Autodesk Fusion 360 part; units mm, degrees
note: some values were not read from the file. Set by a fixed rule: which sketch regions a step uses.
(part 2 of 2)
sketch "Sketch5" plane through (0, 0, 0) normal (0, 0, 1) x (1, 0, 0)
  line L0 (-28.8618, -57.7236) -> (1022.0897, -57.7236)
  line L1 (1022.0897, -57.7236) -> (1022.0897, -272.5388)
  line L2 (1022.0897, -272.5388) -> (-28.8618, -272.5388)
  line L3 (-28.8618, -272.5388) -> (-28.8618, -57.7236)
  line L4 (199.3413, -86.9336) -> (377.0355, -86.9336)
  line L5 (377.0355, -86.9336) -> (377.0355, -237.8519)
  line L6 (377.0355, -237.8519) -> (199.3413, -237.8519)
  line L7 (199.3413, -237.8519) -> (199.3413, -86.9336)
  spline S0 degree 3 poles (267.5473, -188.3142) (266.8998, -187.7866) (266.0771, -187.5231) (265.2567, -187.3679) knots 0 0 0 0 1 1 1 1
  spline S1 degree 3 poles (265.2567, -187.3679) (263.5948, -187.0539) (262.7928, -187.5736) (262.4666, -188.5278) knots 0 0 0 0 1 1 1 1
  spline S2 degree 3 poles (262.4666, -188.5278) (261.4698, -191.4391) (265.1758, -197.3711) (261.7953, -199.3136) knots 0 0 0 0 1 1 1 1
  spline S3 degree 3 poles (261.7953, -199.3136) (261.1984, -199.6568) (260.504, -199.7943) (259.8961, -200.1175) knots 0 0 0 0 1 1 1 1
  spline S4 degree 3 poles (259.8961, -200.1175) (259.2237, -200.4753) (258.6608, -201.082) (258.4703, -201.8196) knots 0 0 0 0 1 1 1 1
  spline S5 degree 3 poles (258.4703, -201.8196) (258.2786, -202.5571) (258.5104, -203.4164) (259.1172, -203.8764) knots 0 0 0 0 1 1 1 1
  spline S6 degree 3 poles (259.1172, -203.8764) (259.5863, -204.2318) (260.201, -204.3188) (260.7876, -204.3681) knots 0 0 0 0 1 1 1 1
  spline S7 degree 3 poles (260.7876, -204.3681) (265.3724, -204.7539) (268.5203, -204.1558) (269.4021, -199.0495) knots 0 0 0 0 1 1 1 1
  spline S8 degree 3 poles (269.4021, -199.0495) (269.9376, -195.955) (270.1658, -192.6087) (268.7102, -189.8258) knots 0 0 0 0 1 1 1 1
  spline S9 degree 3 poles (268.7102, -189.8258) (268.4132, -189.2587) (268.0439, -188.7183) (267.5473, -188.3142) knots 0 0 0 0 1 1 1 1
  spline S10 degree 3 poles (312.6049, -189.9938) (311.9453, -189.4832) (311.1152, -189.2398) (310.2912, -189.1059) knots 0 0 0 0 1 1 1 1
  spline S11 degree 3 poles (310.2912, -189.1059) (308.6233, -188.8345) (307.834, -189.3731) (307.5309, -190.3364) knots 0 0 0 0 1 1 1 1
  spline S12 degree 3 poles (307.5309, -190.3364) (306.6096, -193.2708) (310.4641, -199.1073) (307.1335, -201.135) knots 0 0 0 0 1 1 1 1
  spline S13 degree 3 poles (307.1335, -201.135) (306.5451, -201.4928) (305.855, -201.6486) (305.255, -201.9869) knots 0 0 0 0 1 1 1 1
  spline S14 degree 3 poles (305.255, -201.9869) (304.5917, -202.3612) (304.0452, -202.9825) (303.8736, -203.7249) knots 0 0 0 0 1 1 1 1
  spline S15 degree 3 poles (303.8736, -203.7249) (303.7008, -204.4667) (303.9527, -205.3199) (304.5722, -205.7647) knots 0 0 0 0 1 1 1 1
  spline S16 degree 3 poles (304.5722, -205.7647) (305.0499, -206.108) (305.6663, -206.1792) (306.2542, -206.2132) knots 0 0 0 0 1 1 1 1
  spline S17 degree 3 poles (306.2542, -206.2132) (310.8475, -206.4834) (313.9784, -205.8055) (314.7312, -200.6792) knots 0 0 0 0 1 1 1 1
  spline S18 degree 3 poles (314.7312, -200.6792) (315.1882, -197.5713) (315.3318, -194.2213) (313.8056, -191.4756) knots 0 0 0 0 1 1 1 1
  spline S19 degree 3 poles (313.8056, -191.4756) (313.4946, -190.9163) (313.1118, -190.3851) (312.6049, -189.9938) knots 0 0 0 0 1 1 1 1
  line L8 (341.835, -190.3857) -> (341.2265, -189.7771)
  spline S20 degree 2 poles (341.2265, -189.7771) (340.0429, -189.6524) (339.4051, -189.2252) knots 0 0 0 1 1 1
  spline S21 degree 3 poles (339.4051, -189.2252) (338.7661, -188.7986) (338.1399, -188.2953) (337.3841, -188.1602) knots 0 0 0 0 1 1 1 1
  spline S22 degree 3 poles (337.3841, -188.1602) (337.49, -189.3177) (337.7182, -190.4642) (338.0645, -191.5754) knots 0 0 0 0 1 1 1 1
  spline S23 degree 3 poles (338.0645, -191.5754) (335.808, -191.3916) (334.0183, -189.6548) (332.5413, -187.9387) knots 0 0 0 0 1 1 1 1
  spline S24 degree 3 poles (332.5413, -187.9387) (332.0478, -187.3649) (331.4655, -186.6413) (330.7182, -186.6316) knots 0 0 0 0 1 1 1 1
  spline S25 degree 3 poles (330.7182, -186.6316) (330.6567, -187.1318) (333.484, -192.6695) (332.3241, -192.4103) knots 0 0 0 0 1 1 1 1
  spline S26 degree 2 poles (332.3241, -192.4103) (330.6555, -192.0366) (318.896, -185.9001) knots 0 0 0 1 1 1
  spline S27 degree 2 poles (318.896, -185.9001) (321.626, -194.0418) (319.3658, -193.1856) knots 0 0 0 1 1 1
  spline S28 degree 2 poles (319.3658, -193.1856) (317.1057, -192.3287) (308.1388, -184.2784) knots 0 0 0 1 1 1
  spline S29 degree 2 poles (308.1388, -184.2784) (307.8297, -191.9143) (306.1069, -191.004) knots 0 0 0 1 1 1
  spline S30 degree 2 poles (306.1069, -191.004) (304.3847, -190.093) (295.8189, -180.6435) knots 0 0 0 1 1 1
  spline S31 degree 2 poles (295.8189, -180.6435) (295.1081, -189.6779) (292.2291, -188.0702) knots 0 0 0 1 1 1
  spline S32 degree 2 poles (292.2291, -188.0702) (289.3495, -186.4618) (282.7693, -175.1813) knots 0 0 0 1 1 1
  spline S33 degree 2 poles (282.7693, -175.1813) (288.6101, -163.1796) (279.7388, -164.0821) knots 0 0 0 1 1 1
  spline S34 degree 3 poles (279.7388, -164.0821) (275.6281, -164.5008) (272.1966, -166.0489) (270.29, -169.9241) knots 0 0 0 0 1 1 1 1
  spline S35 degree 3 poles (270.29, -169.9241) (268.8027, -168.3297) (266.5115, -167.639) (264.336, -167.7771) knots 0 0 0 0 1 1 1 1
  spline S36 degree 3 poles (264.336, -167.7771) (262.284, -167.9865) (260.8972, -168.5384) (259.032, -169.4464) knots 0 0 0 0 1 1 1 1
  spline S37 degree 3 poles (259.032, -169.4464) (258.5963, -169.6581) (258.0893, -169.873) (257.6463, -169.6776) knots 0 0 0 0 1 1 1 1
  spline S38 degree 3 poles (257.6463, -169.6776) (257.3554, -169.5498) (257.165, -169.2735) (256.9648, -169.0277) knots 0 0 0 0 1 1 1 1
  spline S39 degree 3 poles (256.9648, -169.0277) (256.2101, -168.0985) (255.1032, -167.4455) (253.9147, -167.3073) knots 0 0 0 0 1 1 1 1
  spline S40 degree 3 poles (253.9147, -167.3073) (252.7135, -167.168) (250.4527, -167.7601) (250.0797, -169.1476) knots 0 0 0 0 1 1 1 1
  spline S41 degree 3 poles (250.0797, -169.1476) (250.5264, -167.4856) (251.1714, -165.1196) (250.4655, -163.4303) knots 0 0 0 0 1 1 1 1
  spline S42 degree 3 poles (250.4655, -163.4303) (250.3365, -163.1212) (250.1187, -162.8479) (249.8479, -162.6264) knots 0 0 0 0 1 1 1 1
  spline S43 degree 3 poles (249.8479, -162.6264) (248.9935, -161.9254) (247.6096, -161.7349) (246.8131, -162.5382) knots 0 0 0 0 1 1 1 1
  spline S44 degree 3 poles (246.8131, -162.5382) (246.185, -163.1717) (246.1564, -164.2086) (246.4528, -165.0503) knots 0 0 0 0 1 1 1 1
  spline S45 degree 3 poles (246.4528, -165.0503) (246.7492, -165.8913) (247.3108, -166.6081) (247.766, -167.3755) knots 0 0 0 0 1 1 1 1
  spline S46 degree 3 poles (247.766, -167.3755) (248.747, -169.0326) (249.6269, -171.6176) (249.0403, -173.5285) knots 0 0 0 0 1 1 1 1
  spline S47 degree 3 poles (249.0403, -173.5285) (248.4969, -175.2969) (246.883, -176.8462) (245.2674, -177.6386) knots 0 0 0 0 1 1 1 1
  spline S48 degree 3 poles (245.2674, -177.6386) (238.2831, -181.0653) (232.6152, -184.0861) (235.577, -186.5007) knots 0 0 0 0 1 1 1 1
  spline S49 degree 3 poles (235.577, -186.5007) (238.5387, -188.9154) (253.3829, -190.6638) (259.2194, -191.9721) knots 0 0 0 0 1 1 1 1
  spline S50 degree 3 poles (259.2194, -191.9721) (265.0559, -193.2793) (270.7872, -196.2271) (282.1925, -198.8687) knots 0 0 0 0 1 1 1 1
  spline S51 degree 3 poles (282.1925, -198.8687) (293.5965, -201.5104) (328.2505, -200.429) (337.1937, -194.9017) knots 0 0 0 0 1 1 1 1
  spline S52 degree 3 poles (337.1937, -194.9017) (339.2347, -193.642) (343.1957, -194.1337) (342.1393, -191.2985) knots 0 0 0 0 1 1 1 1
  line L9 (342.1393, -191.2985) -> (341.835, -190.3857)
  spline S53 degree 3 poles (278.798, -190.7575) (278.1505, -190.2305) (277.3278, -189.967) (276.5074, -189.8118) knots 0 0 0 0 1 1 1 1
  spline S54 degree 3 poles (276.5074, -189.8118) (274.8467, -189.4978) (274.0441, -190.0163) (273.7173, -190.9717) knots 0 0 0 0 1 1 1 1
  spline S55 degree 3 poles (273.7173, -190.9717) (272.7211, -193.8817) (276.4265, -199.8138) (273.0461, -201.7575) knots 0 0 0 0 1 1 1 1
  spline S56 degree 3 poles (273.0461, -201.7575) (272.4491, -202.0995) (271.7554, -202.2382) (271.1468, -202.5614) knots 0 0 0 0 1 1 1 1
  spline S57 degree 3 poles (271.1468, -202.5614) (270.4744, -202.9186) (269.9127, -203.5259) (269.721, -204.2635) knots 0 0 0 0 1 1 1 1
  spline S58 degree 3 poles (269.721, -204.2635) (269.5299, -205.001) (269.7605, -205.8597) (270.3679, -206.3197) knots 0 0 0 0 1 1 1 1
  spline S59 degree 3 poles (270.3679, -206.3197) (270.8365, -206.6757) (271.4517, -206.7628) (272.0383, -206.812) knots 0 0 0 0 1 1 1 1
  spline S60 degree 3 poles (272.0383, -206.812) (276.6231, -207.1979) (279.7711, -206.5991) (280.6535, -201.4934) knots 0 0 0 0 1 1 1 1
  spline S61 degree 3 poles (280.6535, -201.4934) (281.1884, -198.3983) (281.4172, -195.0526) (279.9609, -192.2697) knots 0 0 0 0 1 1 1 1
  spline S62 degree 3 poles (279.9609, -192.2697) (279.664, -191.7026) (279.2946, -191.1616) (278.798, -190.7575) knots 0 0 0 0 1 1 1 1
  spline S63 degree 3 poles (327.0627, -190.6504) (326.4024, -190.1398) (325.5729, -189.897) (324.7496, -189.7625) knots 0 0 0 0 1 1 1 1
  spline S64 degree 3 poles (324.7496, -189.7625) (323.0804, -189.4905) (322.2911, -190.0297) (321.9893, -190.9924) knots 0 0 0 0 1 1 1 1
  spline S65 degree 3 poles (321.9893, -190.9924) (321.0667, -193.9274) (324.9212, -199.7639) (321.5906, -201.7916) knots 0 0 0 0 1 1 1 1
  spline S66 degree 3 poles (321.5906, -201.7916) (321.0034, -202.1494) (320.3121, -202.3058) (319.7133, -202.6435) knots 0 0 0 0 1 1 1 1
  spline S67 degree 3 poles (319.7133, -202.6435) (319.0494, -203.0184) (318.5023, -203.6391) (318.3307, -204.3815) knots 0 0 0 0 1 1 1 1
  spline S68 degree 3 poles (318.3307, -204.3815) (318.1579, -205.1239) (318.4104, -205.9765) (319.0293, -206.4214) knots 0 0 0 0 1 1 1 1
  spline S69 degree 3 poles (319.0293, -206.4214) (319.507, -206.7646) (320.1235, -206.8358) (320.7113, -206.8705) knots 0 0 0 0 1 1 1 1
  spline S70 degree 3 poles (320.7113, -206.8705) (325.3046, -207.14) (328.4367, -206.4615) (329.1895, -201.3352) knots 0 0 0 0 1 1 1 1
  spline S71 degree 3 poles (329.1895, -201.3352) (329.6453, -198.2279) (329.7889, -194.8773) (328.2633, -192.1328) knots 0 0 0 0 1 1 1 1
  spline S72 degree 3 poles (328.2633, -192.1328) (327.9517, -191.5729) (327.569, -191.0411) (327.0627, -190.6504) knots 0 0 0 0 1 1 1 1
  line L10 (614.3667, -86.9336) -> (792.0609, -86.9336)
  line L11 (792.0609, -86.9336) -> (792.0609, -237.8519)
  line L12 (792.0609, -237.8519) -> (614.3667, -237.8519)
  line L13 (614.3667, -237.8519) -> (614.3667, -86.9336)
  spline S73 degree 3 poles (661.9365, -162.4475) (662.7458, -161.7508) (664.0542, -161.9528) (664.8757, -162.6264) knots 0 0 0 0 1 1 1 1
  spline S74 degree 3 poles (664.8757, -162.6264) (665.1434, -162.8479) (665.3626, -163.1212) (665.4903, -163.4303) knots 0 0 0 0 1 1 1 1
  spline S75 degree 3 poles (665.4903, -163.4303) (666.1902, -165.1069) (665.5634, -167.4491) (665.113, -169.1092) knots 0 0 0 0 1 1 1 1
  line L14 (665.113, -169.1092) -> (665.107, -169.147)
  spline S76 degree 3 poles (665.107, -169.147) (665.4782, -167.7601) (667.7419, -167.168) (668.9408, -167.3073) knots 0 0 0 0 1 1 1 1
  spline S77 degree 3 poles (668.9408, -167.3073) (670.1274, -167.4455) (671.2349, -168.0985) (671.9895, -169.0277) knots 0 0 0 0 1 1 1 1
  spline S78 degree 3 poles (671.9895, -169.0277) (672.02, -169.0606) (672.0443, -169.0946) (672.0686, -169.1287) knots 0 0 0 0 1 1 1 1
  spline S79 degree 3 poles (672.0686, -169.1287) (672.2451, -169.3454) (672.4216, -169.5675) (672.6712, -169.6776) knots 0 0 0 0 1 1 1 1
  spline S80 degree 3 poles (672.6712, -169.6776) (673.1154, -169.873) (673.6204, -169.6581) (674.0586, -169.4464) knots 0 0 0 0 1 1 1 1
  spline S81 degree 3 poles (674.0586, -169.4464) (675.9207, -168.5384) (677.3082, -167.9865) (679.359, -167.7771) knots 0 0 0 0 1 1 1 1
  spline S82 degree 3 poles (679.359, -167.7771) (681.5376, -167.639) (683.8257, -168.3297) (685.3166, -169.9241) knots 0 0 0 0 1 1 1 1
  spline S83 degree 3 poles (685.3166, -169.9241) (687.2213, -166.0489) (690.6535, -164.5008) (694.7612, -164.0821) knots 0 0 0 0 1 1 1 1
  spline S84 degree 2 poles (694.7612, -164.0821) (703.6337, -163.1796) (697.7917, -175.1813) knots 0 0 0 1 1 1
  spline S85 degree 2 poles (697.7917, -175.1813) (704.3762, -186.4618) (707.2546, -188.0702) knots 0 0 0 1 1 1
  spline S86 degree 2 poles (707.2546, -188.0702) (710.1329, -189.6779) (710.845, -180.6435) knots 0 0 0 1 1 1
  spline S87 degree 2 poles (710.845, -180.6435) (719.4071, -190.093) (721.1354, -191.004) knots 0 0 0 1 1 1
  spline S88 degree 2 poles (721.1354, -191.004) (722.8576, -191.9143) (723.1618, -184.2784) knots 0 0 0 1 1 1
  spline S89 degree 2 poles (723.1618, -184.2784) (732.1317, -192.3287) (734.3894, -193.1856) knots 0 0 0 1 1 1
  spline S90 degree 2 poles (734.3894, -193.1856) (736.6532, -194.0418) (733.9208, -185.9001) knots 0 0 0 1 1 1
  spline S91 degree 2 poles (733.9208, -185.9001) (745.684, -192.0366) (747.3514, -192.4103) knots 0 0 0 1 1 1
  spline S92 degree 3 poles (747.3514, -192.4103) (748.1181, -192.5825) (747.1323, -190.1982) (746.3959, -188.4304) knots 0 0 0 0 1 1 1 1
  line L15 (746.3959, -188.4304) -> (746.3959, -188.4298)
  line L16 (746.3959, -188.4298) -> (746.3959, -188.4292)
  spline S93 degree 3 poles (746.3959, -188.4292) (746.0308, -187.5353) (745.7204, -186.7995) (745.7448, -186.6316) knots 0 0 0 0 1 1 1 1
  spline S94 degree 3 poles (745.7448, -186.6316) (746.4568, -186.6407) (747.0166, -187.2967) (747.4974, -187.8548) knots 0 0 0 0 1 1 1 1
  line L17 (747.4974, -187.8548) -> (747.5643, -187.9387)
  spline S95 degree 3 poles (747.5643, -187.9387) (749.0431, -189.6548) (750.8322, -191.3916) (753.0899, -191.5754) knots 0 0 0 0 1 1 1 1
  spline S96 degree 3 poles (753.0899, -191.5754) (752.743, -190.4642) (752.5179, -189.3177) (752.4083, -188.1602) knots 0 0 0 0 1 1 1 1
  spline S97 degree 3 poles (752.4083, -188.1602) (753.0473, -188.2746) (753.595, -188.6501) (754.1305, -189.0213) knots 0 0 0 0 1 1 1 1
  spline S98 degree 3 poles (754.1305, -189.0213) (754.2278, -189.0901) (754.3313, -189.1589) (754.4287, -189.2252) knots 0 0 0 0 1 1 1 1
  spline S99 degree 3 poles (754.4287, -189.2252) (754.7391, -189.4321) (755.1772, -189.5684) (755.5423, -189.6536) knots 0 0 0 0 1 1 1 1
  spline S100 degree 3 poles (755.5423, -189.6536) (755.2259, -187.8657) (753.3638, -186.3462) (751.9519, -185.1924) knots 0 0 0 0 1 1 1 1
  spline S101 degree 3 poles (751.9519, -185.1924) (749.9133, -183.5244) (748.8058, -182.6213) (754.6356, -182.7789) knots 0 0 0 0 1 1 1 1
  spline S102 degree 3 poles (754.6356, -182.7789) (754.4165, -180.9618) (752.4205, -180.0301) (750.4002, -179.0851) knots 0 0 0 0 1 1 1 1
  spline S103 degree 3 poles (750.4002, -179.0851) (748.5563, -178.2228) (746.688, -177.3483) (746.116, -175.7807) knots 0 0 0 0 1 1 1 1
  spline S104 degree 3 poles (746.116, -175.7807) (747.3209, -176.5225) (748.3859, -176.0229) (749.463, -175.5166) knots 0 0 0 0 1 1 1 1
  spline S105 degree 3 poles (749.463, -175.5166) (750.5219, -175.0218) (751.5868, -174.521) (752.81, -175.1721) knots 0 0 0 0 1 1 1 1
  spline S106 degree 3 poles (752.81, -175.1721) (752.67, -172.4982) (750.0776, -170.4091) (747.6739, -168.4709) knots 0 0 0 0 1 1 1 1
  spline S107 degree 3 poles (747.6739, -168.4709) (746.7793, -167.7497) (745.9091, -167.0499) (745.2032, -166.3483) knots 0 0 0 0 1 1 1 1
  spline S108 degree 3 poles (745.2032, -166.3483) (744.6008, -165.7513) (743.9861, -165.3229) (743.4262, -164.9292) knots 0 0 0 0 1 1 1 1
  spline S109 degree 3 poles (743.4262, -164.9292) (742.2213, -164.0918) (741.2538, -163.4145) (741.126, -161.6157) knots 0 0 0 0 1 1 1 1
  line L18 (741.126, -161.6157) -> (748.0633, -162.2948)
  spline S110 degree 3 poles (748.0633, -162.2948) (745.2276, -158.6618) (741.0408, -156.1059) (736.5132, -155.2387) knots 0 0 0 0 1 1 1 1
  spline S111 degree 3 poles (736.5132, -155.2387) (735.7282, -155.0896) (734.6937, -154.6442) (734.8945, -153.8738) knots 0 0 0 0 1 1 1 1
  spline S112 degree 3 poles (734.8945, -153.8738) (735.0527, -153.3011) (735.7952, -153.1679) (736.3854, -153.1557) knots 0 0 0 0 1 1 1 1
  spline S113 degree 3 poles (736.3854, -153.1557) (738.844, -153.104) (741.3085, -153.2239) (743.7549, -153.5154) knots 0 0 0 0 1 1 1 1
  spline S114 degree 3 poles (743.7549, -153.5154) (741.6797, -150.9035) (738.2597, -149.7473) (734.9493, -149.3219) knots 0 0 0 0 1 1 1 1
  spline S115 degree 3 poles (734.9493, -149.3219) (733.5131, -149.1369) (732.0587, -149.0645) (730.6104, -148.9921) knots 0 0 0 0 1 1 1 1
  spline S116 degree 3 poles (730.6104, -148.9921) (728.7239, -148.8983) (726.8435, -148.8046) (724.9875, -148.4645) knots 0 0 0 0 1 1 1 1
  spline S117 degree 3 poles (724.9875, -148.4645) (724.6466, -147.5103) (725.955, -146.8512) (726.953, -146.7088) knots 0 0 0 0 1 1 1 1
  spline S118 degree 3 poles (726.953, -146.7088) (729.6246, -146.3291) (732.3386, -146.2323) (735.0345, -146.4204) knots 0 0 0 0 1 1 1 1
  spline S119 degree 3 poles (735.0345, -146.4204) (735.3022, -145.2727) (734.5355, -144.0799) (733.5192, -143.4848) knots 0 0 0 0 1 1 1 1
  spline S120 degree 3 poles (733.5192, -143.4848) (732.5029, -142.8902) (731.2859, -142.7612) (730.1052, -142.6687) knots 0 0 0 0 1 1 1 1
  spline S121 degree 3 poles (730.1052, -142.6687) (726.1497, -142.3571) (722.1699, -142.3042) (718.2022, -142.5129) knots 0 0 0 0 1 1 1 1
  spline S122 degree 3 poles (718.2022, -142.5129) (718.3848, -141.008) (720.2104, -140.4299) (721.6891, -140.0818) knots 0 0 0 0 1 1 1 1
  spline S123 degree 3 poles (721.6891, -140.0818) (723.1679, -139.7349) (724.957, -138.7917) (724.7197, -137.2941) knots 0 0 0 0 1 1 1 1
  spline S124 degree 3 poles (724.7197, -137.2941) (717.8127, -137.3379) (710.918, -138.3548) (704.2971, -140.3033) knots 0 0 0 0 1 1 1 1
  spline S125 degree 3 poles (704.2971, -140.3033) (703.725, -139.2396) (704.7108, -138.0219) (705.648, -137.2582) knots 0 0 0 0 1 1 1 1
  spline S126 degree 3 poles (705.648, -137.2582) (706.5913, -136.4957) (707.6805, -135.4471) (707.3215, -134.2927) knots 0 0 0 0 1 1 1 1
  spline S127 degree 3 poles (707.3215, -134.2927) (703.8285, -133.7791) (700.2989, -134.9305) (697.1162, -136.4494) knots 0 0 0 0 1 1 1 1
  spline S128 degree 3 poles (697.1162, -136.4494) (696.0269, -136.9691) (694.956, -137.5338) (693.8849, -138.0979) knots 0 0 0 0 1 1 1 1
  spline S129 degree 3 poles (693.8849, -138.0979) (691.828, -139.1842) (689.7773, -140.2698) (687.5804, -141.0305) knots 0 0 0 0 1 1 1 1
  spline S130 degree 3 poles (687.5804, -141.0305) (687.7629, -139.3564) (688.262, -137.7176) (689.0409, -136.2236) knots 0 0 0 0 1 1 1 1
  spline S131 degree 3 poles (689.0409, -136.2236) (685.2253, -137.2728) (681.8053, -139.6887) (679.5355, -142.931) knots 0 0 0 0 1 1 1 1
  spline S132 degree 3 poles (679.5355, -142.931) (678.6348, -144.2193) (677.1804, -145.8447) (675.8416, -145.0171) knots 0 0 0 0 1 1 1 1
  line L19 (675.8416, -145.0171) -> (677.0891, -139.7325)
  spline S133 degree 3 poles (677.0891, -139.7325) (676.0485, -139.4775) (675.1235, -140.4043) (674.4724, -141.2538) knots 0 0 0 0 1 1 1 1
  spline S134 degree 3 poles (674.4724, -141.2538) (671.8131, -144.7256) (669.5311, -148.4809) (667.6628, -152.4352) knots 0 0 0 0 1 1 1 1
  spline S135 degree 3 poles (667.6628, -152.4352) (666.7926, -152.7541) (665.9954, -151.753) (665.7885, -150.8469) knots 0 0 0 0 1 1 1 1
  spline S136 degree 3 poles (665.7885, -150.8469) (665.746, -150.6497) (665.7094, -150.4459) (665.6729, -150.2414) knots 0 0 0 0 1 1 1 1
  spline S137 degree 3 poles (665.6729, -150.2414) (665.5451, -149.5032) (665.4112, -148.7529) (664.8513, -148.2825) knots 0 0 0 0 1 1 1 1
  spline S138 degree 3 poles (664.8513, -148.2825) (663.2691, -152.0232) (662.2286, -155.9939) (661.7722, -160.0316) knots 0 0 0 0 1 1 1 1
  line L20 (661.7722, -160.0316) -> (661.7722, -161.1757)
  spline S139 degree 2 poles (661.7722, -161.1757) (661.7356, -161.4939) (661.9365, -162.4475) knots 0 0 0 1 1 1
  line L21 (-8.1714, -88.1507) -> (169.5228, -88.1507)
  line L22 (169.5228, -88.1507) -> (169.5228, -239.069)
  line L23 (169.5228, -239.069) -> (-8.1714, -239.069)
  line L24 (-8.1714, -239.069) -> (-8.1714, -88.1507)
  spline S140 degree 3 poles (115.4575, -199.9921) (115.4946, -201.2524) (115.1788, -202.3387) (114.078, -203.0087) knots 0 0 0 0 1 1 1 1
  spline S141 degree 3 poles (114.078, -203.0087) (113.7682, -203.1973) (113.4299, -203.33) (113.0915, -203.4626) knots 0 0 0 0 1 1 1 1
  spline S142 degree 3 poles (113.0915, -203.4626) (112.7878, -203.5813) (112.4836, -203.7006) (112.2006, -203.8606) knots 0 0 0 0 1 1 1 1
  spline S143 degree 3 poles (112.2006, -203.8606) (111.5367, -204.2355) (110.9896, -204.8562) (110.818, -205.5986) knots 0 0 0 0 1 1 1 1
  spline S144 degree 3 poles (110.818, -205.5986) (110.6452, -206.341) (110.8977, -207.1936) (111.5166, -207.6384) knots 0 0 0 0 1 1 1 1
  spline S145 degree 3 poles (111.5166, -207.6384) (111.9943, -207.9817) (112.6114, -208.0529) (113.1986, -208.0875) knots 0 0 0 0 1 1 1 1
  spline S146 degree 3 poles (113.1986, -208.0875) (117.7919, -208.3571) (120.924, -207.6786) (121.6768, -202.5522) knots 0 0 0 0 1 1 1 1
  spline S147 degree 3 poles (121.6768, -202.5522) (121.8557, -201.3309) (121.9872, -200.0718) (121.9872, -198.8261) knots 0 0 0 0 1 1 1 1
  spline S148 degree 3 poles (121.9872, -198.8261) (125.2745, -198.0862) (127.9557, -197.1849) (129.681, -196.1188) knots 0 0 0 0 1 1 1 1
  spline S149 degree 3 poles (129.681, -196.1188) (130.3485, -195.7068) (131.2224, -195.4816) (132.0579, -195.2668) knots 0 0 0 0 1 1 1 1
  spline S150 degree 3 poles (132.0579, -195.2668) (133.7771, -194.8244) (135.3374, -194.4227) (134.6266, -192.5156) knots 0 0 0 0 1 1 1 1
  line L25 (134.6266, -192.5156) -> (134.5073, -192.1584)
  spline S151 degree 3 poles (134.5073, -192.1584) (135.8345, -192.0811) (138.0022, -191.9082) (138.9131, -191.5711) knots 0 0 0 0 1 1 1 1
  spline S152 degree 2 poles (138.9131, -191.5711) (140.2787, -191.0654) (138.2182, -186.0936) knots 0 0 0 1 1 1
  spline S153 degree 2 poles (138.2182, -186.0936) (142.5121, -187.301) (144.5056, -184.9362) knots 0 0 0 1 1 1
  spline S154 degree 2 poles (144.5056, -184.9362) (146.5211, -182.5458) (135.7889, -175.2555) knots 0 0 0 1 1 1
  spline S155 degree 2 poles (135.7889, -175.2555) (141.7781, -175.4058) (144.1326, -172.9108) knots 0 0 0 1 1 1
  spline S156 degree 2 poles (144.1326, -172.9108) (146.5163, -170.3841) (132.0634, -165.6984) knots 0 0 0 1 1 1
  spline S157 degree 2 poles (132.0634, -165.6984) (139.6477, -164.0109) (140.8611, -160.5696) knots 0 0 0 1 1 1
  spline S158 degree 2 poles (140.8611, -160.5696) (142.0849, -157.0984) (126.9297, -155.0848) knots 0 0 0 1 1 1
  spline S159 degree 2 poles (126.9297, -155.0848) (136.723, -151.3143) (136.5216, -148.1182) knots 0 0 0 1 1 1
  spline S160 degree 2 poles (136.5216, -148.1182) (136.3195, -144.9136) (119.0631, -147.321) knots 0 0 0 1 1 1
  spline S161 degree 2 poles (119.0631, -147.321) (128.4517, -142.0188) (126.9163, -139.5256) knots 0 0 0 1 1 1
  spline S162 degree 2 poles (126.9163, -139.5256) (125.3871, -137.0427) (106.7322, -140.6264) knots 0 0 0 1 1 1
  spline S163 degree 2 poles (106.7322, -140.6264) (119.1501, -132.9339) (116.8486, -129.6459) knots 0 0 0 1 1 1
  spline S164 degree 2 poles (116.8486, -129.6459) (113.7731, -125.2529) (95.0787, -135.7636) knots 0 0 0 1 1 1
  spline S165 degree 2 poles (95.0787, -135.7636) (105.7062, -126.7487) (103.2623, -123.3) knots 0 0 0 1 1 1
  spline S166 degree 2 poles (103.2623, -123.3) (100.8361, -119.8776) (83.8042, -132.5456) knots 0 0 0 1 1 1
  spline S167 degree 2 poles (83.8042, -132.5456) (88.9981, -125.7628) (87.8601, -122.428) knots 0 0 0 1 1 1
  spline S168 degree 2 poles (87.8601, -122.428) (86.7252, -119.0993) (68.9753, -134.4942) knots 0 0 0 1 1 1
  spline S169 degree 2 poles (68.9753, -134.4942) (73.9063, -126.6543) (72.3764, -124.5439) knots 0 0 0 1 1 1
  spline S170 degree 3 poles (72.3764, -124.5439) (71.2561, -122.9982) (62.6848, -131.0328) (57.7757, -135.6346) knots 0 0 0 0 1 1 1 1
  spline S171 degree 3 poles (57.7757, -135.6346) (56.0164, -137.2837) (54.7275, -138.4923) (54.4208, -138.6602) knots 0 0 0 0 1 1 1 1
  spline S172 degree 3 poles (54.4208, -138.6602) (53.9808, -138.9018) (54.2096, -137.9288) (54.5413, -136.5145) knots 0 0 0 0 1 1 1 1
  spline S173 degree 3 poles (54.5413, -136.5145) (55.081, -134.2148) (55.8941, -130.7498) (54.5528, -129.4463) knots 0 0 0 0 1 1 1 1
  spline S174 degree 3 poles (54.5528, -129.4463) (52.8404, -127.782) (47.5114, -138.4917) (44.5314, -144.4816) knots 0 0 0 0 1 1 1 1
  spline S175 degree 3 poles (44.5314, -144.4816) (43.7743, -146.0029) (43.1688, -147.2194) (42.8128, -147.8517) knots 0 0 0 0 1 1 1 1
  spline S176 degree 3 poles (42.8128, -147.8517) (41.9207, -149.4363) (41.4059, -147.5328) (40.7675, -145.1722) knots 0 0 0 0 1 1 1 1
  spline S177 degree 3 poles (40.7675, -145.1722) (40.1633, -142.9383) (39.4482, -140.2948) (38.1983, -139.8086) knots 0 0 0 0 1 1 1 1
  spline S178 degree 3 poles (38.1983, -139.8086) (35.6582, -138.8203) (36.2236, -155.6331) (36.526, -158.6861) knots 0 0 0 0 1 1 1 1
  spline S179 degree 3 poles (36.526, -158.6861) (36.6714, -160.1558) (34.9219, -159.078) (33.1869, -158.0094) knots 0 0 0 0 1 1 1 1
  spline S180 degree 3 poles (33.1869, -158.0094) (31.3238, -156.8623) (29.477, -155.725) (30.0102, -157.7612) knots 0 0 0 0 1 1 1 1
  spline S181 degree 2 poles (30.0102, -157.7612) (31.0407, -161.6984) (34.4235, -167.9007) knots 0 0 0 1 1 1
  spline S182 degree 2 poles (34.4235, -167.9007) (27.8889, -169.6022) (31.2077, -171.6396) knots 0 0 0 1 1 1
  spline S183 degree 3 poles (31.2077, -171.6396) (33.3494, -172.9546) (35.828, -176.5821) (37.3518, -179.054) knots 0 0 0 0 1 1 1 1
  spline S184 degree 3 poles (37.3518, -179.054) (30.5546, -182.3986) (25.1598, -185.35) (28.0642, -187.7178) knots 0 0 0 0 1 1 1 1
  spline S185 degree 3 poles (28.0642, -187.7178) (30.1703, -189.4351) (38.2859, -190.8153) (44.8977, -191.9399) knots 0 0 0 0 1 1 1 1
  spline S186 degree 3 poles (44.8977, -191.9399) (47.5832, -192.3969) (50.0204, -192.8113) (51.7067, -193.1892) knots 0 0 0 0 1 1 1 1
  spline S187 degree 3 poles (51.7067, -193.1892) (52.8739, -193.4503) (54.0374, -193.7777) (55.2429, -194.155) knots 0 0 0 0 1 1 1 1
  line L26 (55.2429, -194.155) -> (55.246, -194.1684)
  spline S188 degree 3 poles (55.246, -194.1684) (55.7778, -196.7139) (56.3298, -199.3538) (54.2826, -200.5307) knots 0 0 0 0 1 1 1 1
  spline S189 degree 3 poles (54.2826, -200.5307) (53.9686, -200.7114) (53.6272, -200.8349) (53.2858, -200.9585) knots 0 0 0 0 1 1 1 1
  spline S190 degree 3 poles (53.2858, -200.9585) (52.9785, -201.0705) (52.6712, -201.1818) (52.3834, -201.3346) knots 0 0 0 0 1 1 1 1
  spline S191 degree 3 poles (52.3834, -201.3346) (51.7109, -201.6924) (51.148, -202.2991) (50.9576, -203.0367) knots 0 0 0 0 1 1 1 1
  spline S192 degree 3 poles (50.9576, -203.0367) (50.7659, -203.7742) (50.9977, -204.6335) (51.6044, -205.0935) knots 0 0 0 0 1 1 1 1
  spline S193 degree 3 poles (51.6044, -205.0935) (52.0736, -205.4489) (52.6883, -205.5359) (53.2749, -205.5852) knots 0 0 0 0 1 1 1 1
  spline S194 degree 3 poles (53.2749, -205.5852) (57.8597, -205.971) (61.0076, -205.3728) (61.8894, -200.2666) knots 0 0 0 0 1 1 1 1
  spline S195 degree 3 poles (61.8894, -200.2666) (62.1006, -199.0477) (62.2637, -197.7892) (62.2953, -196.5423) knots 0 0 0 0 1 1 1 1
  spline S196 degree 3 poles (62.2953, -196.5423) (63.67, -197.006) (65.1494, -197.4886) (66.7693, -197.9785) knots 0 0 0 0 1 1 1 1
  spline S197 degree 3 poles (66.7693, -197.9785) (67.1429, -200.0554) (67.2142, -202.0082) (65.5334, -202.9746) knots 0 0 0 0 1 1 1 1
  spline S198 degree 3 poles (65.5334, -202.9746) (65.2194, -203.1547) (64.8786, -203.2782) (64.5372, -203.4024) knots 0 0 0 0 1 1 1 1
  spline S199 degree 3 poles (64.5372, -203.4024) (64.2299, -203.5137) (63.9226, -203.6251) (63.6341, -203.7785) knots 0 0 0 0 1 1 1 1
  spline S200 degree 3 poles (63.6341, -203.7785) (62.9617, -204.1357) (62.4, -204.743) (62.2083, -205.4805) knots 0 0 0 0 1 1 1 1
  spline S201 degree 3 poles (62.2083, -205.4805) (62.0172, -206.2181) (62.2478, -207.0768) (62.8552, -207.5368) knots 0 0 0 0 1 1 1 1
  spline S202 degree 3 poles (62.8552, -207.5368) (63.3237, -207.8928) (63.939, -207.9798) (64.5256, -208.0291) knots 0 0 0 0 1 1 1 1
  spline S203 degree 3 poles (64.5256, -208.0291) (69.1104, -208.4149) (72.2584, -207.8161) (73.1407, -202.7105) knots 0 0 0 0 1 1 1 1
  spline S204 degree 3 poles (73.1407, -202.7105) (73.3057, -201.7593) (73.4407, -200.7838) (73.5071, -199.8083) knots 0 0 0 0 1 1 1 1
  spline S205 degree 3 poles (73.5071, -199.8083) (73.8911, -199.9014) (74.2818, -199.9939) (74.6797, -200.0858) knots 0 0 0 0 1 1 1 1
  spline S206 degree 3 poles (74.6797, -200.0858) (79.9631, -201.3096) (90.2377, -201.7344) (100.6334, -201.2883) knots 0 0 0 0 1 1 1 1
  spline S207 degree 3 poles (100.6334, -201.2883) (100.4162, -201.7058) (100.0894, -202.0666) (99.6208, -202.352) knots 0 0 0 0 1 1 1 1
  spline S208 degree 3 poles (99.6208, -202.352) (99.3111, -202.5401) (98.9733, -202.6727) (98.6356, -202.8048) knots 0 0 0 0 1 1 1 1
  spline S209 degree 3 poles (98.6356, -202.8048) (98.3313, -202.9241) (98.0264, -203.0433) (97.7423, -203.204) knots 0 0 0 0 1 1 1 1
  spline S210 degree 3 poles (97.7423, -203.204) (97.0789, -203.5783) (96.5325, -204.1996) (96.3609, -204.942) knots 0 0 0 0 1 1 1 1
  spline S211 degree 3 poles (96.3609, -204.942) (96.188, -205.6838) (96.44, -206.537) (97.0595, -206.9818) knots 0 0 0 0 1 1 1 1
  spline S212 degree 3 poles (97.0595, -206.9818) (97.5372, -207.325) (98.1536, -207.3962) (98.7415, -207.4303) knots 0 0 0 0 1 1 1 1
  spline S213 degree 3 poles (98.7415, -207.4303) (103.3348, -207.7005) (106.4657, -207.0226) (107.2185, -201.8962) knots 0 0 0 0 1 1 1 1
  spline S214 degree 3 poles (107.2185, -201.8962) (107.2684, -201.5585) (107.314, -201.2177) (107.3548, -200.8751) knots 0 0 0 0 1 1 1 1
  spline S215 degree 3 poles (107.3548, -200.8751) (110.1595, -200.6481) (112.8943, -200.3542) (115.4575, -199.9921) knots 0 0 0 0 1 1 1 1
  line L27 (406.854, -88.1507) -> (584.5482, -88.1507)
  line L28 (584.5482, -88.1507) -> (584.5482, -239.069)
  line L29 (584.5482, -239.069) -> (406.854, -239.069)
  line L30 (406.854, -239.069) -> (406.854, -88.1507)
  spline S216 degree 3 poles (460.0108, -168.6248) (460.5274, -168.5116) (461.0343, -168.4788) (461.4275, -168.5244) knots 0 0 0 0 1 1 1 1
  spline S217 degree 3 poles (461.4275, -168.5244) (462.6159, -168.6626) (463.7229, -169.3155) (464.4774, -170.2448) knots 0 0 0 0 1 1 1 1
  spline S218 degree 3 poles (464.4774, -170.2448) (464.5042, -170.2776) (464.531, -170.3117) (464.5584, -170.3458) knots 0 0 0 0 1 1 1 1
  spline S219 degree 3 poles (464.5584, -170.3458) (464.7312, -170.5624) (464.9077, -170.7845) (465.159, -170.8947) knots 0 0 0 0 1 1 1 1
  spline S220 degree 3 poles (465.159, -170.8947) (465.602, -171.09) (466.109, -170.8752) (466.5447, -170.6635) knots 0 0 0 0 1 1 1 1
  spline S221 degree 3 poles (466.5447, -170.6635) (468.4099, -169.7555) (469.7967, -169.2036) (471.8487, -168.9942) knots 0 0 0 0 1 1 1 1
  spline S222 degree 3 poles (471.8487, -168.9942) (474.0243, -168.8561) (476.3154, -169.5468) (477.8027, -171.1412) knots 0 0 0 0 1 1 1 1
  spline S223 degree 3 poles (477.8027, -171.1412) (479.7093, -167.266) (483.1408, -165.7178) (487.2515, -165.2992) knots 0 0 0 0 1 1 1 1
  spline S224 degree 3 poles (487.2515, -165.2992) (494.84, -164.5275) (491.6634, -173.1962) (490.5863, -175.7204) knots 0 0 0 0 1 1 1 1
  spline S225 degree 3 poles (490.5863, -175.7204) (491.4498, -176.0016) (492.2787, -176.4154) (493.0576, -176.8852) knots 0 0 0 0 1 1 1 1
  spline S226 degree 3 poles (493.0576, -176.8852) (492.701, -175.9152) (492.5343, -174.8758) (492.5708, -173.8431) knots 0 0 0 0 1 1 1 1
  spline S227 degree 3 poles (492.5708, -173.8431) (492.8318, -173.9538) (493.0929, -174.0646) (493.354, -174.1747) knots 0 0 0 0 1 1 1 1
  spline S228 degree 3 poles (493.354, -174.1747) (493.7264, -174.3323) (494.0988, -174.49) (494.4713, -174.6482) knots 0 0 0 0 1 1 1 1
  spline S229 degree 3 poles (494.4713, -174.6482) (494.4719, -172.9723) (494.4719, -171.2975) (494.4719, -169.6222) knots 0 0 0 0 1 1 1 1
  spline S230 degree 3 poles (494.4719, -169.6222) (495.2386, -170.2016) (496.163, -170.5709) (497.1184, -170.6787) knots 0 0 0 0 1 1 1 1
  spline S231 degree 3 poles (497.1184, -170.6787) (496.2208, -168.9985) (495.6756, -167.1303) (495.5289, -165.231) knots 0 0 0 0 1 1 1 1
  spline S232 degree 3 poles (495.5289, -165.231) (498.4036, -166.63) (501.4019, -167.7741) (504.4775, -168.6443) knots 0 0 0 0 1 1 1 1
  spline S233 degree 3 poles (504.4775, -168.6443) (501.722, -164.5939) (498.526, -160.8428) (494.966, -157.4776) knots 0 0 0 0 1 1 1 1
  spline S234 degree 3 poles (494.966, -157.4776) (499.4716, -157.5043) (503.9749, -157.9042) (508.4148, -158.6703) knots 0 0 0 0 1 1 1 1
  spline S235 degree 3 poles (508.4148, -158.6703) (502.7109, -154.1574) (495.2277, -151.9569) (487.9879, -152.6652) knots 0 0 0 0 1 1 1 1
  spline S236 degree 3 poles (487.9879, -152.6652) (490.0867, -151.8133) (492.16, -150.8956) (494.2017, -149.9128) knots 0 0 0 0 1 1 1 1
  spline S237 degree 3 poles (494.2017, -149.9128) (486.8481, -147.8943) (478.4891, -150.0923) (473.0798, -155.4657) knots 0 0 0 0 1 1 1 1
  spline S238 degree 3 poles (473.0798, -155.4657) (473.4431, -152.978) (474.3504, -150.5718) (475.7185, -148.462) knots 0 0 0 0 1 1 1 1
  spline S239 degree 3 poles (475.7185, -148.462) (470.1162, -150.7404) (465.4876, -155.3142) (463.1423, -160.8891) knots 0 0 0 0 1 1 1 1
  line L31 (463.1423, -160.8891) -> (463.4247, -154.0989)
  spline S240 degree 3 poles (463.4247, -154.0989) (460.2444, -158.0825) (459.847, -163.4242) (460.0108, -168.6248) knots 0 0 0 0 1 1 1 1
  line L32 (821.8795, -88.1507) -> (999.5736, -88.1507)
  line L33 (999.5736, -88.1507) -> (999.5736, -239.069)
  line L34 (999.5736, -239.069) -> (821.8795, -239.069)
  line L35 (821.8795, -239.069) -> (821.8795, -88.1507)
  spline S241 degree 3 poles (860.4549, -183.3881) (859.4995, -183.1739) (858.5015, -183.1708) (857.5583, -183.444) knots 0 0 0 0 1 1 1 1
  spline S242 degree 3 poles (857.5583, -183.444) (856.6454, -183.7094) (855.7204, -184.2351) (856.0125, -185.266) knots 0 0 0 0 1 1 1 1
  spline S243 degree 3 poles (856.0125, -185.266) (856.5541, -187.1683) (857.9599, -188.7085) (859.5482, -189.0712) knots 0 0 0 0 1 1 1 1
  spline S244 degree 3 poles (859.5482, -189.0712) (861.1304, -189.4333) (863.1203, -186.3699) (862.81, -184.9033) knots 0 0 0 0 1 1 1 1
  spline S245 degree 3 poles (862.81, -184.9033) (862.6274, -184.0489) (861.4408, -183.6084) (860.4549, -183.3881) knots 0 0 0 0 1 1 1 1
  spline S246 degree 3 poles (903.6127, -167.0639) (901.8175, -166.8954) (899.9554, -167.1491) (898.367, -167.992) knots 0 0 0 0 1 1 1 1
  spline S247 degree 3 poles (898.367, -167.992) (896.7787, -168.8354) (895.4825, -170.3014) (895.0444, -172.0473) knots 0 0 0 0 1 1 1 1
  spline S248 degree 3 poles (895.0444, -172.0473) (894.9105, -172.567) (894.9166, -173.237) (895.3852, -173.4974) knots 0 0 0 0 1 1 1 1
  spline S249 degree 3 poles (895.3852, -173.4974) (895.6529, -173.6441) (895.9755, -173.6015) (896.2798, -173.5534) knots 0 0 0 0 1 1 1 1
  spline S250 degree 3 poles (896.2798, -173.5534) (898.72, -173.1658) (899.6146, -173.3191) (900.4057, -175.7533) knots 0 0 0 0 1 1 1 1
  spline S251 degree 3 poles (900.4057, -175.7533) (900.7161, -176.7026) (903.7952, -173.2467) (903.917, -172.94) knots 0 0 0 0 1 1 1 1
  spline S252 degree 3 poles (903.917, -172.94) (904.3551, -171.8221) (904.3673, -170.5831) (904.2821, -169.3837) knots 0 0 0 0 1 1 1 1
  spline S253 degree 3 poles (904.2821, -169.3837) (904.2273, -168.5682) (904.1178, -167.7072) (903.6127, -167.0639) knots 0 0 0 0 1 1 1 1
  spline S254 degree 3 poles (882.9771, -174.2837) (881.6321, -174.0238) (880.2873, -175.1472) (879.9647, -176.7927) knots 0 0 0 0 1 1 1 1
  spline S255 degree 3 poles (879.9647, -176.7927) (879.6483, -178.4382) (880.482, -179.9827) (881.8208, -180.2425) knots 0 0 0 0 1 1 1 1
  spline S256 degree 3 poles (881.8208, -180.2425) (883.1657, -180.503) (884.5106, -179.379) (884.8331, -177.7335) knots 0 0 0 0 1 1 1 1
  spline S257 degree 3 poles (884.8331, -177.7335) (885.1495, -176.088) (884.3219, -174.5441) (882.9771, -174.2837) knots 0 0 0 0 1 1 1 1
  spline S258 degree 3 poles (874.3236, -173.2765) (873.1613, -173.0514) (871.9928, -174.0256) (871.7129, -175.4527) knots 0 0 0 0 1 1 1 1
  spline S259 degree 3 poles (871.7129, -175.4527) (871.4391, -176.8809) (872.1572, -178.2203) (873.3256, -178.4461) knots 0 0 0 0 1 1 1 1
  spline S260 degree 3 poles (873.3256, -178.4461) (874.4879, -178.6719) (875.6563, -177.697) (875.9362, -176.2699) knots 0 0 0 0 1 1 1 1
  spline S261 degree 3 poles (875.9362, -176.2699) (876.2101, -174.8429) (875.492, -173.5023) (874.3236, -173.2765) knots 0 0 0 0 1 1 1 1
extrude "Extrude11" add sketch "Sketch5" along normal blind 2 separate body contours S73 S74 S75 L14 S76 S77 S78 S79 S80 S81 S82 S83 S84 S85 S86 S87 S88 S89 S90 S91 S92 S93 S94 L17 S95 S96 S97 S98 S99 S100 S101 S102 S103 S104 S105 S106 S107 S108 S109 L18 S110 S111 S112 S113 S114 S115 S116 S117 S118 S119 S120 S121 S122 S123 S124 S125 S126 S127 S128 S129 S130 S131 S132 L19 S133 S134 S135 S136 S137 S138 L20 S139 makes body 8
sketch "Sketch6" plane through (0, 0, 0) normal (0, 0, 1) x (1, 0, 0)
  ellipse E0 centre (-190.4061, 30.5401) end of major axis (-123.1622, 30.5401) minor radius 54.7687
  point P0 (-123.1622, 30.5401)
extrude "Extrude12" add sketch "Sketch6" along normal blind 1 separate body makes body 9
